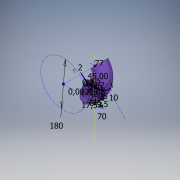
# Autodesk Inventor part: DriveChainEnclosureV3
Saved by Autodesk Inventor 2019.1 (Build 231200000, 200)
## iProperties
Created: 2018-07-04
Part Number: DriveChainEnclosureV3
Material: Generisch
Document SubType Name: Modeling
Designer: JochenAlt
Density: 1 g/cm^3
Appearance: Vorgabe
Author: JochenAlt
Autodesk Inventor part; units mm, degrees
ref_plane "YZ Plane" through (0, 0, 0) normal (1, 0, 0) x (0, 1, 0)
ref_plane "XZ Plane" through (0, 0, 0) normal (0, 1, 0) x (-1, 0, 0)
sketch "Enclosure" plane through (0, 0, 0) normal (0, 1, 0) x (-1, 0, 0)
  line L0 (35, 0) -> (-35, 0) construction
  circle A0 centre (26.215, 0) radius 8.785 construction
  circle A1 centre (-26.215, 0) radius 8.785 construction
  circle A2 centre (125, 0) radius 90 construction
  line L1 (125, 0) -> (0, 125) construction
  line L2 (0, 125) -> (-122.2765, 2.7235) construction
  line L3 (0, -133) -> (0, 168) construction
  line L4 (26.5, 27.7037) -> (26.5, 52.7037)
  line L5 (54.4472, 70.5528) -> (53.033, 71.967)
  line L6 (35, 0) -> (125, 0) construction
  line L7 (26.5, 52.7037) -> (25.8117, 54.5816)
  line L8 (0, 48) -> (0, 50)
  line L9 (0, 50) -> (0, 52)
  arc A3 (-54.4472, 70.5528) -> (26.5, 52.7037) centre (0, 125) ccw
  arc A4 (26.5, 52.7037) -> (54.4472, 70.5528) centre (0, 125) ccw
  line L10 (24, 51.8358) -> (24, 53.9437)
  line L11 (26.6877, 52.7728) -> (25.9945, 54.6488)
  line L12 (24, 27.7037) -> (24, 51.8358)
  arc A5 (-53.033, 71.967) -> (-41.0959, 62.2614) centre (0, 125) ccw
  line L13 (25.8117, 54.5816) -> (25.1234, 56.4594)
  line L14 (25.9945, 54.6488) -> (25.3013, 56.5249)
  arc A6 (17.3, 56.1399) -> (26.3752, 59.0807) centre (0, 125) ccw
  line L15 (17.3, 54.0796) -> (17.3, 56.1399)
  arc A7 (0, 52) -> (25.3013, 56.5249) centre (0, 125) ccw
  arc A8 (-40, 63.9345) -> (0, 52) centre (0, 125) ccw
  line L16 (-40, 63.9345) -> (-41.0959, 62.2614)
  line L17 (26.3752, 59.0807) -> (17.3, 59.0807)
  line L18 (17.3, 59.0807) -> (17.3, 56.1399)
  line L19 (27.8611, 55.367) -> (26.3752, 59.0807)
  line L20 (18.3935, -4) -> (-18.3935, -4) construction
  line L21 (18.3935, 4) -> (-18.3935, 4) construction
  line L22 (23.8, 51.7705) -> (23.8, 53.8764)
  arc A9 (-38.9041, 65.6075) -> (0, 54) centre (0, 125) ccw
  line L23 (-40, 63.9345) -> (-38.9041, 65.6075)
  line L24 (0, 52) -> (0, 54)
  arc A10 (-41.0959, 62.2614) -> (0, 50) centre (0, 125) ccw
  arc A11 (16.2, 51.7705) -> (53.033, 71.967) centre (0, 125) ccw
  arc A12 (0, 50) -> (16.2, 51.7705) centre (0, 125) ccw
  line L25 (-53.033, 71.967) -> (-60.1041, 79.0381)
  line L26 (-60.1041, 79.0381) -> (-61.5183, 77.6238)
  line L27 (-54.4472, 70.5528) -> (-51.877, 67.9826)
  line L28 (-54.377, 70.4826) -> (-61.5183, 77.6238)
  line L29 (-54.377, 70.4826) -> (-51.877, 67.9826)
  line L30 (-26.5, 27.7037) -> (-26.5, 52.7037)
  line L31 (-24, 27.7037) -> (-24, 51.8358)
  line L32 (15.706, 7.8686) -> (15.706, 8.048) construction
  spline S0 degree 4 poles (-26.5, 27.7037) (-26.5, 21.2487) (-24.3745, 7.5876) (0, 11.344) (24.3745, 7.5876) (26.5, 21.2487) (26.5, 27.7037) knots 0 0 0 0 0 0.375 0.625 1 1 1 1 1
  spline S1 degree 4 poles (-24, 27.7037) (-24, 22.1495) (-23.294, 10.0475) (0, 13.9135) (23.294, 10.0475) (24, 22.1495) (24, 27.7037) knots 0 0 0 0 0 0.375 0.625 1 1 1 1 1
  line L33 (-26.5, 27.7037) -> (-24, 27.7037) construction
  line L34 (-24, 51.8358) -> (-24, 53.9437)
  line L35 (-26.5, 52.7037) -> (-25.8117, 54.5816)
  point P0 (-24, 10.048)
  point P1 (24, 10.048)
  point P2 (0, 0)
  point P3 (0, 5)
  point P4 (-21.443, 13.3129)
  point P5 (0, 9.5)
  point P6 (21.443, 13.3129)
  point P7 (-20.3244, 15.4656)
  point P8 (20.3244, 15.4656)
  point P9 (0, 12)
  dimension "d42" = 180
  dimension "d31" = 70
  dimension "d32" = 17.57
  dimension "d106" = 0
  dimension "d672" = 0.2
  dimension "d1173" = 2
  dimension "d1175" = 40
  dimension "d1225" = 2
  dimension "d1238" = 8
  dimension "d1249" = 0.2
  dimension "d1259" = 23.8
  dimension "d1274" = 2
  dimension "d1281" = 45
  dimension "d1282" = 10
  dimension "d1496" = 2
  dimension "d1580" = 17.3
  dimension "d1627" = 77
  dimension "d1628" = 2
  dimension "d1648" = 1
  dimension "d1685" = 25
  dimension "d1686" = 26.5
  dimension "d1687" = 2.5
  dimension "d1688" = 9.5
  dimension "d1689" = 2.5
  constraints: 70 end point, 44 point on circle, 12 centre point, 11 vertical, 10 coincident, 7 point on line, 6 collinear, 6 parallel, 5 horizontal alignment, 5 perpendicular, 4 horizontal, 3 line through centre, 3 tangent, 1 equal radius, 1 midpoint, 22 other
  measures "d31" distance of L0.end L0.start
  measures "d32" diameter of A0
  measures "d106" distance between parallel lines of L6 L0
  measures "d672" distance of L11.start L4.end
  measures "d1173" radial gap between concentric circles of A6 A7
  measures "d1225" distance of L19.start L11.end
  measures "d1238" distance between parallel lines of L20 L21
  measures "d1249" distance between parallel lines of L10 L22
  measures "d1259" distance of the line from the sketch origin of L22
  measures "d1274" radial gap between concentric circles of A8 A10
  measures "d1281" angle to the sketch x axis of L2
  measures "d1282" distance between parallel lines of L2 L26
  measures "d1496" distance of L5.start L5.end
  measures "d1580" distance of the line from the sketch origin of L15
  measures "d1627" distance between parallel lines of L1 L29
  measures "d1628" radial gap between concentric circles of A9 A8
  measures "d1648" distance from line of L21 point (0, 5)
  measures "d1685" distance of L30.start L30.end
  measures "d1686" distance of the line from the sketch origin of L30
  measures "d1687" distance between parallel lines of L31 L30
  measures "d1688" distance of point (0, 0) point (0, 9.5)
  measures "d1689" distance of point (0, 9.5) point (0, 12)
revolve "Umdrehung1" add sketch "Enclosure" angle 90 about axis through (-125, 0, 0) along (0.7071068, 0, 0.7071068) and the other way 30 contours S0 L30 A3 L31 S1 L12 L4
ref_plane "Arbeitsebene52" through (0, 0, 5) normal (0, 0, 1) x (1, 0, 0)
sketch "OmniwheelBearing" plane through (0, 0, 5) normal (0, 0, 1) x (1, 0, 0)
  circle A0 centre (0, 0) radius 4.15
  circle A1 centre (0, 0) radius 5.65
  circle A2 centre (0, 0) radius 3.65
  line L0 (-7.91, 0) -> (7.91, 0) construction
  line L1 (0, -7.91) -> (0, 7.91) construction
  dimension "d26" = 8.3
  dimension "d27" = 1.5
  dimension "d28" = 0.5
  constraints: 3 centre point, 2 coincident
  measures "d26" diameter of A0
  measures "d27" radial gap between concentric circles of A1 A0
  measures "d28" radial gap between concentric circles of A0 A2
extrude "Extrusion254" add sketch "OmniwheelBearing" along normal up to next contours A1
chamfer "Fase24" distance 4 angle 45 2 edges at (-5.4949, 1.3149, 9.5605) (5.4949, -1.3148, 9.5601)
extrude "Extrusion258" cut sketch "OmniwheelBearing" along normal through all contours A0 | A1 | A2
extrude "Extrusion264" add sketch "OmniwheelBearing" along normal blind 6 contours A0 | A1
extrude "Extrusion265" add sketch "OmniwheelBearing" along normal blind 3 from surface at 6 contours A1
sketch "BeltDriveBearing" plane through (0, 0, 5) normal (0, 0, 1) x (1, 0, 0)
  arc A0 (-0.0634, 34.9813) -> (-11.4443, 33.0563) centre (-5.2199, 30.8617) ccw construction
  arc A1 (15.3255, 23.6177) -> (-22.2401, 17.264) centre (-5.2199, 30.8617) ccw construction
  arc A2 (-5.1565, -4.1196) -> (6.2244, -2.1946) centre (0, 0) ccw construction
  line L0 (-11.4443, 33.0563) -> (-20.5453, 7.244) construction
  line L1 (-22.2401, 17.264) -> (-5.1565, -4.1196) construction
  line L2 (15.3255, 23.6177) -> (6.2244, -2.1946) construction
  line L3 (-0.0634, 34.9813) -> (17.0202, 13.5977) construction
  arc A3 (-20.5453, 7.244) -> (17.0202, 13.5977) centre (0, 0) ccw construction
  arc A4 (-13.4781, 13.2208) -> (-13.4781, 13.2208) centre (-5.2199, 30.8617) ccw
  circle A5 centre (-5.2199, 30.8617) radius 4.1
  arc A6 (-1.2054, 34.7661) -> (-10.1667, 33.4863) centre (-5.2199, 30.8617) ccw
  circle A7 centre (-5.2199, 30.8617) radius 3.1
  arc A8 (-10.1667, 33.4863) -> (-1.2054, 34.7661) centre (-5.2199, 30.8617) ccw
  line L4 (0, 0) -> (-3.709, 21.9287) construction
  line L5 (0, 72.1922) -> (0, -41.3305) construction
  line L6 (-45.4778, 0) -> (60.5368, 0) construction
  point P0 (45.3919, 0)
  point P1 (45.3919, 0)
  dimension "d891" = 43.57
  dimension "d892" = 6.6
  dimension "d893" = 31.3
  dimension "d1081" = 8.2
  dimension "d1082" = 1.5
  dimension "d1087" = 1
  dimension "d1625" = 99.6
  constraints: 14 point on circle, 11 coincident, 10 end point, 9 centre point, 8 tangent, 2 equal radius, 1 point on line, 2 other
  measures "d891" diameter of A1
  measures "d892" radius of A0
  measures "d893" distance of point (0, 0) A0.centre
  measures "d1081" diameter of A5
  measures "d1082" radial gap between concentric circles of A6 A5
  measures "d1087" radial gap between concentric circles of A5 A7
  measures "d1625" angle of L6 L4
ref_plane "Arbeitsebene55" through (0, 0, 16) normal (0, 0, 1) x (1, 0, 0)
extrude "Extrusion260" add sketch "BeltDriveBearing" along normal blind 1.4 from surface at 11 contours A5 | A8 A6
extrude "Extrusion261" add sketch "BeltDriveBearing" along normal blind 0.5 from surface at 12.4 contours A5 | A8 A6
extrude "Extrusion262" add sketch "BeltDriveBearing" along normal blind 3 from surface at 12.9 contours A8 A6
sketch "Screws" plane through (0, 0, 0) normal (0, 0, 1) x (1, 0, 0)
  line L0 (0, 31.5) -> (0, -31.5) construction
  circle A0 centre (0, 0) radius 22.5 construction
  circle A1 centre (20.3919, -9.5089) radius 1.2
  circle A2 centre (20.3919, 9.5089) radius 1.2
  circle A3 centre (-20.3919, -9.5089) radius 1.2
  circle A4 centre (20.3919, -9.5089) radius 2.15 construction
  circle A5 centre (20.3919, 9.5089) radius 2.15 construction
  circle A6 centre (-20.3919, -9.5089) radius 2.15 construction
  arc A7 (20.3919, -5.5089) -> (20.3919, -13.5089) centre (20.3919, -9.5089) ccw
  arc A8 (20.3919, 13.5089) -> (20.3919, 5.5089) centre (20.3919, 9.5089) ccw
  arc A9 (-20.3919, -13.5089) -> (-20.3919, -5.5089) centre (-20.3919, -9.5089) ccw
  line L1 (17.9188, 9.7253) -> (19.3427, 11.7589)
  line L2 (19.3427, 11.7589) -> (21.8159, 11.5425)
  line L3 (21.8159, 11.5425) -> (22.8651, 9.2925)
  line L4 (22.8651, 9.2925) -> (21.4411, 7.2589)
  line L5 (21.4411, 7.2589) -> (18.968, 7.4753)
  line L6 (18.968, 7.4753) -> (17.9188, 9.7253)
  line L7 (-17.9188, -9.7253) -> (-19.3427, -11.7589)
  line L8 (-19.3427, -11.7589) -> (-21.8159, -11.5425)
  line L9 (-21.8159, -11.5425) -> (-22.8651, -9.2925)
  line L10 (-22.8651, -9.2925) -> (-21.4411, -7.2589)
  line L11 (-21.4411, -7.2589) -> (-18.968, -7.4753)
  line L12 (-18.968, -7.4753) -> (-17.9188, -9.7253)
  line L13 (-48.7231, 0) -> (48.7231, 0) construction
  circle A10 centre (-20.3919, -9.5089) radius 2.5
  circle A11 centre (20.3919, 9.5089) radius 2.5
  circle A12 centre (20.3919, -9.5089) radius 2.5
  line L14 (20.3919, -13.5089) -> (32.2879, -13.5089)
  line L15 (20.3919, 5.5089) -> (34.5637, 5.5089)
  line L16 (20.3919, 13.5089) -> (32.2879, 13.5089)
  line L17 (20.3919, -5.5089) -> (34.5637, -5.5089)
  arc A13 (32.2879, -13.5089) -> (34.5637, -5.5089) centre (0, 0) ccw
  arc A14 (34.5637, 5.5089) -> (32.2879, 13.5089) centre (0, 0) ccw
  arc A15 (-34.5637, -5.5089) -> (-32.2879, -13.5089) centre (0, 0) ccw
  circle A16 centre (20.3919, 9.5089) radius 1.5
  circle A17 centre (20.3919, -9.5089) radius 1.5
  circle A18 centre (-20.3919, -9.5089) radius 1.5
  line L18 (20.3919, 9.5089) -> (0, 0) construction
  line L19 (0, 0) -> (-20.3919, -9.5089) construction
  line L20 (-20.3919, -13.5089) -> (-32.2879, -13.5089)
  line L21 (-20.3919, -5.5089) -> (-34.5637, -5.5089)
  line L22 (0, 0) -> (-20.3919, 9.5089) construction
  circle A19 centre (-20.3919, 9.5089) radius 1.5
  circle A20 centre (-20.3919, 9.5089) radius 1.2
  circle A21 centre (-20.3919, 9.5089) radius 2.5
  circle A22 centre (-20.3919, 9.5089) radius 2.15 construction
  line L23 (-18.968, 7.4753) -> (-21.4411, 7.2589)
  line L24 (-21.4411, 7.2589) -> (-22.8651, 9.2925)
  line L25 (-22.8651, 9.2925) -> (-21.8159, 11.5425)
  line L26 (-21.8159, 11.5425) -> (-19.3427, 11.7589)
  line L27 (-19.3427, 11.7589) -> (-17.9188, 9.7253)
  line L28 (-17.9188, 9.7253) -> (-18.968, 7.4753)
  arc A23 (-20.3919, 5.5089) -> (-20.3919, 13.5089) centre (-20.3919, 9.5089) ccw
  line L29 (-20.3919, 13.5089) -> (-32.2879, 13.5089)
  arc A24 (-32.2879, 13.5089) -> (-34.5637, 5.5089) centre (0, 0) ccw
  line L30 (-20.3919, 5.5089) -> (-34.5637, 5.5089)
  line L31 (20.3919, -9.5089) -> (0, 0) construction
  line L32 (18.968, -7.4753) -> (21.4411, -7.2589)
  line L33 (21.4411, -7.2589) -> (22.8651, -9.2925)
  line L34 (22.8651, -9.2925) -> (21.8159, -11.5425)
  line L35 (21.8159, -11.5425) -> (19.3427, -11.7589)
  line L36 (19.3427, -11.7589) -> (17.9188, -9.7253)
  line L37 (17.9188, -9.7253) -> (18.968, -7.4753)
  point P0 (18.4434, 8.6003)
  point P1 (-18.4434, -8.6003)
  point P2 (-18.4434, 8.6003)
  point P3 (18.4434, -8.6003)
  dimension "d1208" = 4.3
  dimension "d1205" = 2.4
  dimension "d1206" = 45
  dimension "d1209" = 8
  dimension "d1216" = 5
  dimension "d1618" = 0.3
  dimension "d1701" = 35
  dimension "d1702" = 25
  dimension "d1703" = 25
  dimension "d1704" = 25
  dimension "d1705" = 25
  dimension "d655" = 29.1
  dimension "d656" = 39.1
  dimension "d1258" = 2.01
  dimension "d1574" = 45.98
  dimension "d1132" = 41.5
  dimension "d1227" = 30.2
  dimension "d1228" = 2
  dimension "d1250" = 2
  dimension "d1140" = 1
  dimension "d1141" = 7
  dimension "d1142" = 7
  dimension "d1275" = 19
  dimension "d1150" = 2.4
  dimension "d1151" = 6
  dimension "d1153" = 3
  dimension "d1620" = 2
  dimension "d1294" = 13
  dimension "d1295" = 10
  dimension "d1351" = 15.3
  dimension "d1298" = 3.5
  dimension "d1299" = 2
  dimension "d1301" = 5
  dimension "d1451" = 5
  dimension "d1499" = 5
  dimension "d1501" = 1.5
  dimension "d1508" = 0.2
  dimension "d1522" = 25.2
  dimension "d1525" = 2
  dimension "d1527" = 2
  dimension "d1540" = 2
  dimension "d1541" = 8
  dimension "d1592" = 25.776
  dimension "d1530" = 4.5
  dimension "d1531" = 2.5
  dimension "d1533" = 8
  dimension "d1424" = 2
  dimension "d1436" = 30
  dimension "d1449" = 115
  dimension "d1450" = 75
  constraints: 72 end point, 22 coincident, 21 centre point, 20 point on circle, 15 equal radius, 8 tangent, 6 parallel, 4 midpoint, 4 point on line, 2 horizontal, 65 other
  measures "d1205" diameter of A3
  measures "d1206" diameter of A0
  measures "d1209" diameter of A9
  measures "d1216" diameter of A10
  measures "d1618" radial gap between concentric circles of A18 A3
  measures "d1701" radius of A14
  measures "d1702" angle to the sketch x axis of L19
  measures "d1703" angle to the sketch x axis of L22
  measures "d1704" angle to the sketch x axis of L18
  measures "d1705" angle to the sketch x axis of L31
ref_plane "Arbeitsebene56" through (0, 0, 45) normal (0, 0, 1) x (1, 0, 0)
extrude "Extrusion267" add sketch "Screws" along normal blind 100 from surface at 45 separate body contours L17 A13 L14 A7 | L16 A14 L15 A8 | L20 A15 L21 A9 | L1 L2 L3 L4 L5 L6 | L7 L8 L9 L10 L11 L12 | A10 | A11 | A12 | A16 | A17 | A21 | L23 L24 L25 L26 L27 L28 | L30 A24 L29 A23 | L32 L33 L34 L35 L36 L37
revolve "Umdrehung51" cut sketch "Enclosure" angle 360 about axis through (-125, 0, 0) along (0.7071068, 0, 0.7071068) keep common part bodies 2 contours L12 S1 L31 A3
extrude "Extrusion268" cut sketch "Screws" along normal blind 2 from surface at 45 contours L1 L2 L3 L4 L5 L6 | L7 L8 L9 L10 L11 L12 | A16 | A17 | A18 | A19 | L23 L24 L25 L26 L27 L28 | L32 L33 L34 L35 L36 L37 bodies 2
combine bodies "Kombinieren47" operation type add bodies to combine 1 2
revolve "Umdrehung50" add sketch "Enclosure" angle 25 about axis through (-125, 0, 0) along (0.7071068, 0, 0.7071068) and the other way 25 bodies 1 contours A3 L10 A11 L7 | L35 A10 L34 A3
equation "\"d851\" = 60deg"
equation "\"Skizze50_Pitch\" = 2.30909"
